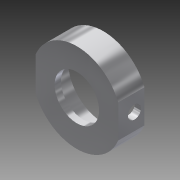
# Autodesk Inventor part: Pneumatic Connector -Shaft Side Cover
Saved by Autodesk Inventor 2013 (Build 170138000, 138)
## iProperties
Created: 2013-06-08
Part Number: Pneumatic Connector -Shaft Side Cover
Material: Generic
Document SubType Name: Modeling
Designer: mvarma
Density: 1 g/cm^3
Author: mvarma
Autodesk Inventor part; units mm, degrees
ref_plane "YZ Plane" through (0, 0, 0) normal (1, 0, 0) x (0, 1, 0)
ref_plane "XZ Plane" through (0, 0, 0) normal (0, 1, 0) x (-1, 0, 0)
ref_plane "XY Plane" through (0, 0, 0) normal (0, 0, 1) x (1, 0, 0)
sketch "Sketch1" plane through (0, 0, 0) normal (0, 0, 1) x (1, 0, 0)
  circle A0 centre (0, 0) radius 11.1125
  circle A1 centre (0, 0) radius 6.35
  circle A2 centre (0, 0) radius 8.7313
  dimension "d0" = 22.225
  dimension "d1" = 12.7
  dimension "d34" = 2.3813
  dimension "d35" = 2.3813
  constraints: 3 centre point, 3 coincident
  measures "d0" diameter of A0
  measures "d1" diameter of A1
  measures "d34" radial gap between concentric circles of A2 A1
  measures "d35" radial gap between concentric circles of A0 A2
extrude "Extrusion3" add sketch "Sketch1" along normal blind 4.9784 contours A0
sketch "Sketch2" plane through (0, 0, 4.9784) normal (0, 0, 1) x (1, 0, 0)
  circle A0 centre (0, 0) radius 11.1125 projected
  circle A1 centre (0, 0) radius 5.5563
  dimension "d36" = 11.1125
  constraints: 1 centre point, 1 coincident
  measures "d36" diameter of A1
extrude "Extrusion4" add sketch "Sketch2" along normal blind 1.5875
sketch "Sketch3" plane through (0, 0, 0) normal (1, 0, 0) x (0, 1, 0)
  line L0 (-8.7313, 4.9784) -> (8.7313, 4.9784) projected
  line L1 (8.7313, 0) -> (-8.7313, 0) projected
  line L2 (0, 0) -> (0, 4.9784) construction
  point P0 (0, 2.4892)
  constraints: 2 end point, 2 midpoint, 1 perpendicular
hole "Hole2" at (0, 0, 2.4892) direction (-1, 0, 0) diameter 3.2766 end through all clearance for "Flat Head Machine Screw (82)" size "#4" standard "Ansi Unified Screw Threads"
sketch "Sketch4" plane through (0, 0, 0) normal (0, 0, -1) x (-1, 0, 0)
  circle A0 centre (0, 0) radius 11.1125 projected
  line L0 (0, 0) -> (-11.1125, 0) construction
  line L1 (-10.3187, 4.1244) -> (-10.3187, -4.1244)
  circle A1 centre (0, 0) radius 7.9375 construction
  point P0 (-7.9375, 0)
  point P1 (-10.3187, 0)
  dimension "d30" = 15.875
  dimension "d29" = 0.7937
  constraints: 4 end point, 3 point on circle, 1 coincident, 1 horizontal, 1 horizontal alignment, 1 midpoint, 1 perpendicular, 1 point on line, 2 other
  measures "d29" distance from line of L0.end L1
extrude "Extrusion5" cut sketch "Sketch4" against normal through all contours L1 A0 picked at (-10.5166, 0.7)
mirror "Mirror1" about plane through (0, 0, 0) normal (1, 0, 0) of "Hole2", "Extrusion5"
equation "\"d34\" = d35"
body "Solid2"
